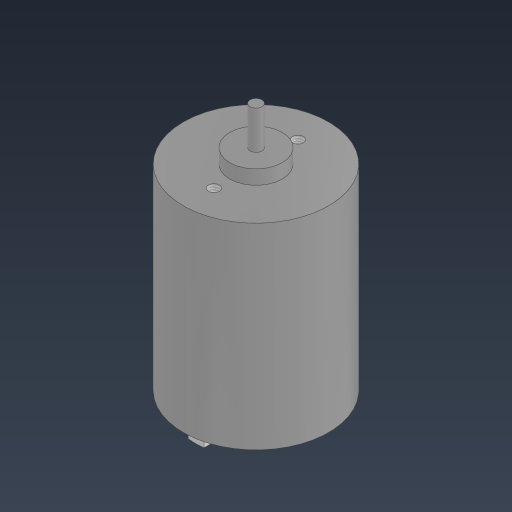
# Autodesk Inventor part: rs385
Saved by Autodesk Inventor 2023 (Build 270158000, 158)
## iProperties
Created: 2025-03-30
Part Number: rs385
Material: Generic
Document SubType Name: Modeling
Designer: szymo
Density: 3.04857 g/cm^3
Appearance: Default
Mass: 70 g
Surface Area: 47.9525 cm^2
Volume: 22.9616 cm^3
Author: szymo
Autodesk Inventor part; units mm, degrees
ref_plane "YZ Plane" through (0, 0, 0) normal (1, 0, 0) x (0, 1, 0)
ref_plane "XZ Plane" through (0, 0, 0) normal (0, 1, 0) x (-1, 0, 0)
ref_plane "XY Plane" through (0, 0, 0) normal (0, 0, 1) x (1, 0, 0)
sketch "Sketch1" plane through (0, 0, 0) normal (0, 1, 0) x (-1, 0, 0)
  circle A0 centre (0, 0) radius 13.85
  dimension "d0" = 27.7
  constraints: 1 centre point, 1 coincident
  measures "d0" diameter of A0
extrude "Extrusion1" add sketch "Sketch1" along normal blind 37.4
sketch "Sketch2" plane through (0, 37.4, 0) normal (0, 1, 0) x (1, 0, 0)
  circle A0 centre (0, 0) radius 5
  circle A1 centre (0, 0) radius 1.15
  circle A2 centre (0, 0) radius 8
  line L0 (0, -8) -> (0, 8)
  dimension "d3" = 10
  dimension "d6" = 2.3
  dimension "d9" = 16
  constraints: 6 coincident, 3 centre point, 2 end point, 2 point on circle, 1 midpoint, 1 vertical
  measures "d3" diameter of A0
  measures "d6" diameter of A1
  measures "d9" diameter of A2
extrude "Extrusion2" add sketch "Sketch2" along normal blind 2.7 contours A0 L0 A1 | L0 A1 A0 | L0 A1 | A1 L0
extrude "Extrusion3" add sketch "Sketch2" along normal blind 10 contours L0 A1 | A1 L0
hole "Hole1" at (0, 37.4, 8) at (0, 37.4, -8) direction (0, -1, 0) diameter 2.1129 depth 7.8 thread size "M2.6x0.45" class "6H" standard "ISO Metric profile"
sketch "Sketch3" plane through (0, 0, 0) normal (0, -1, 0) x (1, 0, 0)
  circle A0 centre (0, 0) radius 5
  dimension "d17" = 10
  constraints: 1 centre point, 1 coincident
  measures "d17" diameter of A0
extrude "Extrusion4" add sketch "Sketch3" along normal blind 3
sketch "Sketch4" plane through (0, 0, 0) normal (0, -1, 0) x (1, 0, 0)
  line L0 (-12.0122, 7.6623) -> (12.8258, 7.6623) construction
  line L1 (12.8258, 7.6623) -> (12.8258, -7.5309) construction
  line L2 (12.8258, -7.5309) -> (-12.0122, -7.5309) construction
  line L3 (-12.0122, -7.5309) -> (-12.0122, 7.6623) construction
  point P0 (0, 0)
  constraints: 2 other
sketch "Sketch5" plane through (0, 0, 0) normal (0, -1, 0) x (1, 0, 0)
  circle A0 centre (0, 8) radius 1.0564 projected
  circle A1 centre (0, -8) radius 1.0564 projected
  circle A2 centre (0, 0) radius 5 projected
  circle A3 centre (0, 0) radius 13.85 projected
  circle A4 centre (0, 0) radius 1.15 projected
  circle A5 centre (0, 0) radius 11.5
  circle A6 centre (0, 0) radius 7.5
  line L0 (1.5, 11.4018) -> (1.5, 7.3485)
  line L1 (-1.5, 11.4018) -> (-1.5, 7.3485)
  line L2 (1.5, -7.3485) -> (1.5, -11.4018)
  line L3 (-1.5, -7.3485) -> (-1.5, -11.4018)
  dimension "d20" = 23
  dimension "d21" = 4
  dimension "d22" = 1.5
  dimension "d23" = 1.5
  dimension "d24" = 1.5
  constraints: 8 end point, 8 point on circle, 2 centre point, 2 coincident, 2 parallel, 2 point on line, 1 vertical
  measures "d20" diameter of A5
  measures "d21" radial gap between concentric circles of A5 A6
  measures "d22" distance from line of L1 point (0, 0)
  measures "d23" distance from line of point (0, 0) L0
  measures "d24" distance from line of point (0, 0) L2
extrude "Extrusion5" add sketch "Sketch5" along normal up to surface (3 mm away) contours A0 A6 | A0 A6 L1 A5 L0 | A6 A1 L2 A5 L3 | A6 A1 picked at (0.0328, 8.0133) picked at (0.0328, -8.0133)
equation "\"d23\" = d22"
equation "\"d24\" = d22"
body "Solid1"
